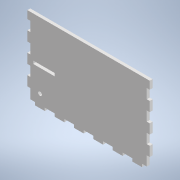
# Autodesk Inventor part: back
Saved by Autodesk Inventor 2022 (Build 260153070, 153G)
## iProperties
Created: 2022-05-11
Part Number: back
Material: Generic
Document SubType Name: Modeling
Designer: Jeanette Guo
Density: 1 g/cm^3
Appearance: Default
Author: Jeanette Guo
Autodesk Inventor part; units mm, degrees
ref_plane "YZ Plane" through (0, 0, 0) normal (1, 0, 0) x (0, 1, 0)
ref_plane "XZ Plane" through (0, 0, 0) normal (0, 1, 0) x (-1, 0, 0)
ref_plane "XY Plane" through (0, 0, 0) normal (0, 0, 1) x (1, 0, 0)
ref_plane "Work Plane2" through (0, 0, 0) normal (0, 0, 1) x (1, 0, 0)
sketch "Sketch2" plane through (0, 0, 0) normal (0, 0, 1) x (1, 0, 0)
  line L0 (-13, 0) -> (-13, 3) projected
  line L1 (-13, 3) -> (-10, 3) projected
  line L2 (103, 0) -> (103, 3) projected
  line L3 (100, 3) -> (103, 3) projected
  line L4 (103, 8) -> (-13, 8)
  line L5 (-10, 0) -> (-10, 3) projected
  line L6 (-10, 3) -> (0, 3) projected
  line L7 (100, 0) -> (100, 3) projected
  line L8 (90, 3) -> (100, 3) projected
  line L9 (90, 3) -> (0, 3)
  line L10 (0, 0) -> (90, 0)
  line L11 (0, 0) -> (0, 3) projected
  line L12 (90, 0) -> (90, 3) projected
  line L13 (90, 3) -> (90, 0)
  line L14 (0, 3) -> (0, 0)
  line L15 (45, 0) -> (45, -20) construction
  line L16 (-15.0005, 0) -> (-15.0005, -10)
  line L17 (-15.0005, -10) -> (-18.0005, -10)
  line L18 (-15.0005, -20) -> (-18.0005, -20)
  line L19 (-15.0005, -20) -> (-15.0005, -30)
  line L20 (-15.0005, -30) -> (-18.0005, -30)
  line L21 (-15.0005, -40) -> (-18.0005, -40)
  line L22 (-15.0005, -50) -> (-18.0005, -50)
  line L23 (-15.0005, -60) -> (-18.0005, -60)
  line L24 (-18.0005, -10) -> (-18.0005, -20)
  line L25 (-18.0005, -30) -> (-18.0005, -40)
  line L26 (-18.0005, -50) -> (-18.0005, -60)
  line L27 (-15.0005, -40) -> (-15.0005, -50)
  line L28 (90, -73) -> (90, -70)
  line L29 (80, -73) -> (70, -73)
  line L30 (60, -73) -> (50, -73)
  line L31 (45, -70) -> (45, -47.72) construction
  line L32 (80, -73) -> (80, -70)
  line L33 (70, -73) -> (70, -70)
  line L34 (60, -73) -> (60, -70)
  line L35 (90, -70) -> (80, -70)
  line L36 (80, -73) -> (70, -73)
  line L37 (70, -70) -> (60, -70)
  line L38 (-10, -73) -> (0, -73)
  line L39 (0, -73) -> (0, -70)
  line L40 (10, -73) -> (20, -73)
  line L41 (10, -73) -> (10, -70)
  line L42 (20, -73) -> (20, -70)
  line L43 (30, -73) -> (30, -70)
  line L44 (0, -70) -> (10, -70)
  line L45 (20, -70) -> (30, -70)
  line L46 (60, -73) -> (50, -73)
  line L47 (50, -73) -> (50, -70)
  line L48 (50, -70) -> (45, -70)
  line L49 (45, -70) -> (40, -70)
  line L50 (40, -70) -> (40, -73)
  line L51 (30, -73) -> (40, -73)
  line L52 (50, -73) -> (77.2719, -73)
  line L53 (60, -73) -> (50, -73)
  line L54 (45, -70) -> (40, -70)
  line L55 (40, -73) -> (30, -73)
  line L56 (30, -70) -> (20, -70)
  line L57 (10, -70) -> (0, -70)
  line L58 (20, -73) -> (10, -73)
  line L59 (0, -73) -> (12.7281, -73)
  line L60 (-18, 8) -> (-13, 8)
  line L61 (-15.0005, 0) -> (-18, 0)
  line L62 (-15.0005, -60) -> (-15.0005, -70)
  line L63 (-18, -50) -> (-18, -60)
  line L64 (-18, -30) -> (-18, -40)
  line L65 (-18, 8) -> (-18, 0)
  line L66 (-18, -10) -> (-18, -20)
  line L67 (105.0005, 0) -> (105.0005, -10)
  line L68 (108.0005, -10) -> (108.0005, -20)
  line L69 (105.0005, -10) -> (108.0005, -10)
  line L70 (105.0005, -20) -> (108.0005, -20)
  line L71 (105.0005, -20) -> (105.0005, -30)
  line L72 (105.0005, -30) -> (108.0005, -30)
  line L73 (108.0005, -30) -> (108.0005, -40)
  line L74 (105.0005, -40) -> (108.0005, -40)
  line L75 (105.0005, -40) -> (105.0005, -50)
  line L76 (105.0005, -50) -> (108.0005, -50)
  line L77 (108.0005, -50) -> (108.0005, -60)
  line L78 (105.0005, -60) -> (108.0005, -60)
  line L79 (108, 8) -> (103, 8)
  line L80 (105.0005, 0) -> (108, 0)
  line L81 (105.0005, -60) -> (105.0005, -70)
  line L82 (108, -50) -> (108, -60)
  line L83 (108, -30) -> (108, -40)
  line L84 (108, 8) -> (108, 0)
  line L85 (108, -10) -> (108, -20)
  line L86 (100, -73) -> (90, -73)
  line L87 (0, -73) -> (-10, -73)
  line L88 (-10, -73) -> (-10, -70)
  line L89 (-10, -70) -> (-15.0005, -70)
  line L90 (-13, -73) -> (-10, -73)
  line L91 (100, -73) -> (98, -73)
  line L92 (90, -70) -> (100, -70)
  line L93 (100, -70) -> (100, -73)
  line L94 (105.0005, -70) -> (100, -70)
  dimension "d39" = 10
  dimension "d42" = 10
  constraints: 170 end point, 32 symmetric about line, 28 perpendicular, 25 parallel, 20 point on line, 8 vertical, 7 collinear, 3 horizontal, 1 midpoint, 1 other
  measures "d39" distance of L38.end L38.start
  measures "d42" distance of L28.end L92.end
extrude "Extrusion1" add sketch "Sketch2" along normal blind 3 contours L79 L84 L80 L67 L69 L68 L70 L71 L72 L73 L74 L75 L76 L77 L78 L81 L94 L92 L35 L32 L29 L33 L37 L34 L30 L47 L48 L49 L50 L51 L43 L45 L42 L40 L41 L44 L39 L38 L88 L89 L62 L23 L26 L22 L27 L21 L25 L20 L19 L18 L24 L17 L16 L61 L65 L60 L4 | L93 L86 L28 L92 | L12 L10 L11 L9
sketch "Sketch3" plane through (0, 0, 3) normal (0, 0, 1) x (1, 0, 0)
  line L0 (0, -70) -> (10, -70) projected
  line L1 (-15.0005, -40) -> (-15.0005, -50) projected
  line L2 (-9.2505, -64.25) -> (7.7495, -64.25)
  line L3 (7.7495, -64.25) -> (7.7495, -55.25)
  line L4 (7.7495, -55.25) -> (-9.2505, -55.25)
  line L5 (-9.2505, -55.25) -> (-9.2505, -64.25)
  line L6 (16.5, -70) -> (16.5, 3) projected
  line L7 (13.5, 3) -> (13.5, -70) projected
  circle A0 centre (-5.0005, -60) radius 2
  line L8 (-15.0005, -60) -> (-15.0005, -70) projected
  line L9 (-15.0005, -70) -> (-10, -70) projected
  point P0 (0, 0)
  dimension "d57" = 17
  dimension "d58" = 9
  dimension "d59" = 5.75
  dimension "d60" = 5.75
  dimension "d61" = 4
  dimension "d62" = 10
  dimension "d63" = 10
  constraints: 8 end point, 2 parallel, 1 centre point, 1 horizontal, 1 perpendicular
  measures "d57" distance of L3.end L4.end
  measures "d58" distance of L2.end L3.end
  measures "d59" distance between parallel lines of L2 L0
  measures "d60" distance between parallel lines of L5 L1
  measures "d61" diameter of A0
  measures "d62" distance from line of L8 A0.centre
  measures "d63" distance from line of L9 A0.centre
extrude "Extrusion2" cut sketch "Sketch3" against normal blind 10 contours A0
sketch "Sketch4" plane through (0, 0, 3) normal (0, 0, 1) x (1, 0, 0)
  line L0 (-12, -37) -> (10, -37)
  line L1 (10, -37) -> (10, -34)
  line L2 (10, -34) -> (-12, -34)
  line L3 (-12, -34) -> (-12, -37)
  line L4 (108, 8) -> (-18, 8) projected
  line L5 (-18, -30) -> (-18, -40) projected
  dimension "d51" = 22
  dimension "d52" = 3
  dimension "d53" = 45
  dimension "d54" = 6
  constraints: 8 end point, 2 parallel, 1 horizontal, 1 perpendicular
  measures "d51" distance of L2.end L1.end
  measures "d52" distance of L1.end L0.end
  measures "d53" distance between parallel lines of L0 L4
  measures "d54" distance between parallel lines of L5 L3
extrude "Extrusion3" cut sketch "Sketch4" against normal blind 10
body "Solid1"
